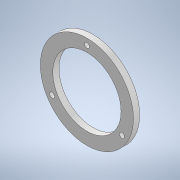
# Autodesk Inventor part: Tractor_Mobile_2
Saved by Autodesk Inventor 2022 (Build 260153070, 153G)
## iProperties
Created: 2022-03-05
Part Number: Tractor_Mobile_2
Material: Generic
Document SubType Name: Modeling
Designer: a laptop
Density: 1 g/cm^3
Appearance: Default
Author: a laptop
Autodesk Inventor part; units mm, degrees
ref_plane "YZ Plane" through (0, 0, 0) normal (1, 0, 0) x (0, 1, 0)
ref_plane "XZ Plane" through (0, 0, 0) normal (0, 1, 0) x (-1, 0, 0)
ref_plane "XY Plane" through (0, 0, 0) normal (0, 0, 1) x (1, 0, 0)
sketch "Sketch1" plane through (0, 0, 0) normal (0, 0, 1) x (1, 0, 0)
  circle A0 centre (0, 0) radius 55.075
  circle A1 centre (0, 0) radius 75.075
  circle A2 centre (0, 65.075) radius 4
  circle A3 centre (-56.3566, -32.5375) radius 4
  circle A4 centre (56.3566, -32.5375) radius 4
  line L0 (0, 65.075) -> (-56.3566, -32.5375) construction
  line L1 (-56.3566, -32.5375) -> (56.3566, -32.5375) construction
  line L2 (56.3566, -32.5375) -> (0, 65.075) construction
  line L3 (0, 65.075) -> (0, 55.075) construction
  line L4 (-56.3566, -32.5375) -> (-47.6963, -27.5375) construction
  line L5 (56.3566, -32.5375) -> (47.6963, -27.5375) construction
  dimension "d0" = 20
  dimension "d1" = 110.15
  dimension "d7" = 8
  dimension "d8" = 10
  constraints: 12 end point, 5 centre point, 4 equal length, 3 line through centre, 3 point on circle, 2 coincident, 2 equal radius, 1 vertical
  measures "d0" radial gap between concentric circles of A1 A0
  measures "d1" diameter of A0
  measures "d7" diameter of A2
  measures "d8" distance of L0.start L3.end
extrude "Extrusion1" add sketch "Sketch1" along normal blind 12
body "Solid1"
